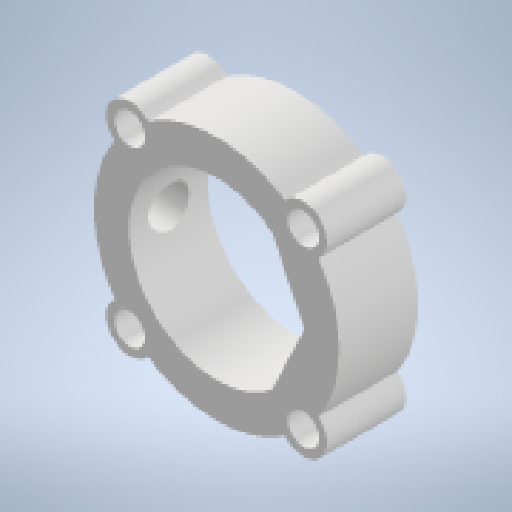
# Autodesk Inventor part: marker_holder
Saved by Autodesk Inventor 2024 (Build 280153000, 153)
## iProperties
Created: 2026-02-08
Part Number: marker_holder
Material: Generic
Document SubType Name: Modeling
Designer: SEMEN
Density: 1 g/cm^3
Appearance: Default
Author: SEMEN
Autodesk Inventor part; units mm, degrees
ref_plane "YZ Plane" through (0, 0, 0) normal (1, 0, 0) x (0, 1, 0)
ref_plane "XZ Plane" through (0, 0, 0) normal (0, 1, 0) x (-1, 0, 0)
ref_plane "XY Plane" through (0, 0, 0) normal (0, 0, 1) x (1, 0, 0)
sketch "Sketch1" plane through (0, 0, 0) normal (0, 0, 1) x (1, 0, 0)
  circle A0 centre (84.6636, 36.1746) radius 1.1933 projected
  circle A1 centre (104.4626, 36.1746) radius 1.1933 projected
  circle A2 centre (104.4626, 16.3756) radius 1.1933 projected
  circle A3 centre (84.6636, 16.3756) radius 1.1933 projected
  circle A4 centre (94.5631, 26.2751) radius 10 projected
  circle A5 centre (94.5631, 26.2751) radius 14
  arc A6 (106.175, 34.0958) -> (102.3838, 37.887) centre (104.4626, 36.1746) ccw
  arc A7 (86.7424, 37.887) -> (82.9512, 34.0958) centre (84.6636, 36.1746) ccw
  arc A8 (82.9512, 18.4544) -> (86.7424, 14.6632) centre (84.6636, 16.3756) ccw
  arc A9 (102.3838, 14.6632) -> (106.175, 18.4544) centre (104.4626, 16.3756) ccw
  line L0 (80.5631, 26.2751) -> (108.5631, 26.2751) construction
  line L1 (104.5631, 26.2751) -> (100.935, 18.568)
  line L2 (104.5631, 26.2751) -> (100.935, 33.9822)
  circle A10 centre (94.0631, 26.2751) radius 9.5 construction
  point P0 (0, 0)
  dimension "d0" = 4
  dimension "d1" = 1.5
  dimension "d2" = 1.5
  dimension "d3" = 1.5
  dimension "d4" = 1.5
  dimension "d7" = 19
  constraints: 11 point on circle, 6 end point, 5 centre point, 2 point on line, 2 tangent, 1 horizontal, 1 midpoint, 1 symmetric about line, 12 other
  measures "d1" radial gap between concentric circles of A1 A6
  measures "d2" radial gap between concentric circles of A0 A7
  measures "d3" radial gap between concentric circles of A3 A8
  measures "d4" radial gap between concentric circles of A2 A9
  measures "d7" diameter of A10
extrude "Extrusion1" add sketch "Sketch1" along normal blind 9 contours A0 A5 | A0 A5 A1 A2 A3 | A5 A0 | A0 A5 A7 | A6 A5 A1 | A5 A3 A8 | A5 A1 | A1 A5 | A5 A3 | A3 A5 | A5 A2 A9 | A5 A2 | A2 A5 | L2 A4 | A4 L1
hole "Hole1" at (104.4626, 16.3756, 0) at (84.6636, 16.3756, 0) at (84.6636, 36.1746, 0) at (104.4626, 36.1746, 0) direction (0, 0, 1) diameter 3.5 end through all clearance for "Countersunk Head GOST 12876-67" size "M3" standard "GOST"
sketch "Sketch2" plane through (0, 0, 0) normal (1, 0, 0) x (0, 1, 0)
  line L0 (34.0958, 0) -> (18.4544, 0) projected
  line L1 (18.4544, 0) -> (18.4544, 9) projected
  line L2 (34.0958, 9) -> (18.4544, 9) projected
  line L3 (34.0958, 0) -> (34.0958, 9) projected
  line L4 (26.2751, 0) -> (26.2751, 9) projected
  point P0 (0, 0)
  point P1 (26.2751, 4.5)
  constraints: 1 midpoint
hole "Hole2" at (0, 26.2751, 4.5) direction (1, 0, 0) diameter 4.6 depth 87.5 tip angle 118
body "Solid1"
